Autodesk Inventor part; units mm, degrees
(part 3 of 3)
sketch "Sketch16" plane through (0, 0, 5) normal (0, 0, 1) x (1, 0, 0)
  circle A0 centre (-2.0556, -8.0514) radius 2.05 projected
  circle A1 centre (-5.9738, -25.7804) radius 2.05 projected
  circle A2 centre (11.7552, -29.6986) radius 2.05 projected
  circle A3 centre (15.6735, -11.9696) radius 2.05 projected
  circle A4 centre (-7.3556, -16.1775) radius 1.55 projected
  circle A5 centre (17.0553, -21.5725) radius 1.55 projected
  circle A6 centre (2.1523, -31.0805) radius 1.55 projected
  circle A7 centre (7.5473, -6.6695) radius 1.55 projected
  line L0 (-8.9194, -96.699) -> (-12.8137, -111.6638) projected
  arc A8 (-16.3595, -112.3464) -> (-12.8137, -111.6638) centre (-14.7493, -111.1602) ccw projected
  arc A9 (-16.3595, -112.3464) -> (-18.9305, -109.3855) centre (-36.0848, -126.8778) ccw projected
  arc A10 (-19.7333, -106.4881) -> (-18.9305, -109.3855) centre (-16.83, -107.2436) ccw projected
  line L1 (-19.7333, -106.4881) -> (-18.513, -101.7988) projected
  arc A11 (-16.9119, -99.2479) -> (-18.513, -101.7988) centre (-13.6742, -103.058) ccw projected
  arc A12 (-16.9119, -99.2479) -> (-12.3264, -94.8408) centre (-50.585, -59.6232) ccw projected
  arc A13 (-8.9194, -96.699) -> (-12.3264, -94.8408) centre (-10.8549, -96.1953) ccw projected
  arc A14 (-68.172, -108.5588) -> (-61.3963, -110.4869) centre (-50.585, -59.6232) ccw projected
  arc A15 (-60.0679, -113.4218) -> (-61.3963, -110.4869) centre (-61.8121, -112.4432) ccw projected
  arc A16 (-60.0679, -113.4218) -> (-62.0734, -117.8863) centre (-36.0848, -126.8778) ccw projected
  arc A17 (-65.5871, -118.4003) -> (-62.0734, -117.8863) centre (-63.9634, -117.2324) ccw projected
  line L2 (-65.5871, -118.4003) -> (-70.472, -111.6088) projected
  arc A18 (-68.172, -108.5588) -> (-70.472, -111.6088) centre (-68.8484, -110.441) ccw projected
  circle A19 centre (-16.1129, -136.1039) radius 2.05 projected
  circle A20 centre (-26.8587, -106.9059) radius 2.05 projected
  circle A21 centre (-56.0568, -117.6516) radius 2.05 projected
  circle A22 centre (-45.311, -146.8497) radius 2.05 projected
  circle A23 centre (-43.6086, -47.5396) radius 2.1 projected
  circle A24 centre (-50.585, -18.9546) radius 2.1 projected
  circle A25 centre (-57.5615, -47.5396) radius 2.1 projected
  circle A26 centre (-85.8051, -39.2889) radius 2.1 projected
  circle A27 centre (-64.538, -59.6232) radius 2.1 projected
  circle A28 centre (-85.8051, -79.9575) radius 2.1 projected
  circle A29 centre (-57.5615, -71.7068) radius 2.1 projected
  circle A30 centre (-50.585, -100.2918) radius 2.1 projected
  circle A31 centre (-43.6086, -71.7068) radius 2.1 projected
  circle A32 centre (-15.365, -79.9575) radius 2.1 projected
  circle A33 centre (-15.365, -39.2889) radius 2.1 projected
  circle A34 centre (-36.6321, -59.6232) radius 2.1 projected
  line L3 (-44.13, -38.9303) -> (-49.053, -44.7973) projected
  arc A35 (-52.1171, -44.7973) -> (-49.053, -44.7973) centre (-50.585, -43.5117) ccw projected
  line L4 (-52.1171, -44.7973) -> (-57.0401, -38.9303) projected
  arc A36 (-55.2842, -34.0514) -> (-57.0401, -38.9303) centre (-54.742, -37.0019) ccw projected
  arc A37 (-45.8859, -34.0514) -> (-55.2842, -34.0514) centre (-50.585, -59.6232) ccw projected
  arc A38 (-44.13, -38.9303) -> (-45.8859, -34.0514) centre (-46.4281, -37.0019) ccw projected
  line L5 (-65.2781, -43.6865) -> (-62.6586, -50.8834) projected
  arc A39 (-64.1907, -53.5371) -> (-62.6586, -50.8834) centre (-64.538, -51.5674) ccw projected
  line L6 (-64.1907, -53.5371) -> (-71.7331, -54.867) projected
  arc A40 (-75.0805, -50.9068) -> (-71.7331, -54.867) centre (-72.2541, -51.9126) ccw projected
  arc A41 (-70.3813, -42.7677) -> (-75.0805, -50.9068) centre (-50.585, -59.6232) ccw projected
  arc A42 (-65.2781, -43.6865) -> (-70.3813, -42.7677) centre (-68.0971, -44.7125) ccw projected
  line L7 (-71.7331, -64.3793) -> (-64.1907, -65.7093) projected
  arc A43 (-62.6586, -68.3629) -> (-64.1907, -65.7093) centre (-64.538, -67.6789) ccw projected
  line L8 (-62.6586, -68.3629) -> (-65.2781, -75.5599) projected
  arc A44 (-70.3813, -76.4787) -> (-65.2781, -75.5599) centre (-68.0971, -74.5338) ccw projected
  arc A45 (-75.0805, -68.3395) -> (-70.3813, -76.4787) centre (-50.585, -59.6232) ccw projected
  arc A46 (-71.7331, -64.3793) -> (-75.0805, -68.3395) centre (-72.2541, -67.3338) ccw projected
  line L9 (-57.0401, -80.316) -> (-52.1171, -74.449) projected
  arc A47 (-49.053, -74.449) -> (-52.1171, -74.449) centre (-50.585, -75.7346) ccw projected
  line L10 (-49.053, -74.449) -> (-44.13, -80.316) projected
  arc A48 (-45.8859, -85.195) -> (-44.13, -80.316) centre (-46.4281, -82.2444) ccw projected
  arc A49 (-55.2842, -85.195) -> (-45.8859, -85.195) centre (-50.585, -59.6232) ccw projected
  arc A50 (-57.0401, -80.316) -> (-55.2842, -85.195) centre (-54.742, -82.2444) ccw projected
  line L11 (-35.892, -75.5599) -> (-38.5115, -68.3629) projected
  arc A51 (-36.9794, -65.7093) -> (-38.5115, -68.3629) centre (-36.6321, -67.6789) ccw projected
  line L12 (-36.9794, -65.7093) -> (-29.437, -64.3793) projected
  arc A52 (-26.0896, -68.3395) -> (-29.437, -64.3793) centre (-28.916, -67.3338) ccw projected
  arc A53 (-30.7888, -76.4787) -> (-26.0896, -68.3395) centre (-50.585, -59.6232) ccw projected
  arc A54 (-35.892, -75.5599) -> (-30.7888, -76.4787) centre (-33.073, -74.5338) ccw projected
  line L13 (-29.437, -54.867) -> (-36.9794, -53.5371) projected
  arc A55 (-38.5115, -50.8834) -> (-36.9794, -53.5371) centre (-36.6321, -51.5674) ccw projected
  line L14 (-38.5115, -50.8834) -> (-35.892, -43.6865) projected
  arc A56 (-30.7888, -42.7677) -> (-35.892, -43.6865) centre (-33.073, -44.7125) ccw projected
  arc A57 (-26.0896, -50.9068) -> (-30.7888, -42.7677) centre (-50.585, -59.6232) ccw projected
  arc A58 (-29.437, -54.867) -> (-26.0896, -50.9068) centre (-28.916, -51.9126) ccw projected
  arc A59 (-83.4142, -91.845) -> (-62.0753, -104.165) centre (-50.585, -59.6232) ccw projected
  arc A60 (-83.0768, -85.9345) -> (-83.4142, -91.845) centre (-80.5595, -89.0431) ccw projected
  line L15 (-83.0768, -85.9345) -> (-78.075, -81.8841) projected
  arc A61 (-74.0235, -82.1373) -> (-78.075, -81.8841) centre (-76.1871, -84.2156) ccw projected
  arc A62 (-74.0235, -82.1373) -> (-58.3636, -91.1786) centre (-50.585, -59.6232) ccw projected
  arc A63 (-56.1186, -94.5607) -> (-58.3636, -91.1786) centre (-59.0817, -94.0914) ccw projected
  line L16 (-56.1186, -94.5607) -> (-57.1254, -100.9175) projected
  arc A64 (-62.0753, -104.165) -> (-57.1254, -100.9175) centre (-61.0762, -100.2918) ccw projected
  arc A65 (-39.0948, -104.165) -> (-17.7559, -91.845) centre (-50.585, -59.6232) ccw projected
  arc A66 (-44.0447, -100.9175) -> (-39.0948, -104.165) centre (-40.0939, -100.2918) ccw projected
  line L17 (-44.0447, -100.9175) -> (-45.0515, -94.5607) projected
  arc A67 (-42.8065, -91.1786) -> (-45.0515, -94.5607) centre (-42.0884, -94.0914) ccw projected
  arc A68 (-42.8065, -91.1786) -> (-27.1466, -82.1373) centre (-50.585, -59.6232) ccw projected
  arc A69 (-23.0951, -81.8841) -> (-27.1466, -82.1373) centre (-24.983, -84.2156) ccw projected
  line L18 (-23.0951, -81.8841) -> (-18.0933, -85.9345) projected
  arc A70 (-17.7559, -91.845) -> (-18.0933, -85.9345) centre (-20.6106, -89.0431) ccw projected
  arc A71 (-6.2656, -71.9432) -> (-6.2656, -47.3031) centre (-50.585, -59.6232) ccw projected
  arc A72 (-11.5529, -74.6062) -> (-6.2656, -71.9432) centre (-10.1194, -70.8719) ccw projected
  line L19 (-11.5529, -74.6062) -> (-17.5615, -72.2997) projected
  arc A73 (-19.368, -68.6644) -> (-17.5615, -72.2997) centre (-16.4864, -69.499) ccw projected
  arc A74 (-19.368, -68.6644) -> (-19.368, -50.5819) centre (-50.585, -59.6232) ccw projected
  arc A75 (-17.5615, -46.9466) -> (-19.368, -50.5819) centre (-16.4864, -49.7474) ccw projected
  line L20 (-17.5615, -46.9466) -> (-11.5529, -44.6401) projected
  arc A76 (-6.2656, -47.3031) -> (-11.5529, -44.6401) centre (-10.1194, -48.3745) ccw projected
  arc A77 (-17.7559, -27.4014) -> (-39.0948, -15.0814) centre (-50.585, -59.6232) ccw projected
  arc A78 (-18.0933, -33.3119) -> (-17.7559, -27.4014) centre (-20.6106, -30.2033) ccw projected
  line L21 (-18.0933, -33.3119) -> (-23.0951, -37.3622) projected
  arc A79 (-27.1466, -37.109) -> (-23.0951, -37.3622) centre (-24.983, -35.0308) ccw projected
  arc A80 (-27.1466, -37.109) -> (-42.8065, -28.0678) centre (-50.585, -59.6232) ccw projected
  arc A81 (-45.0515, -24.6857) -> (-42.8065, -28.0678) centre (-42.0884, -25.155) ccw projected
  line L22 (-45.0515, -24.6857) -> (-44.0447, -18.3288) projected
  arc A82 (-39.0948, -15.0814) -> (-44.0447, -18.3288) centre (-40.0939, -18.9546) ccw projected
  arc A83 (-62.0753, -15.0814) -> (-83.4142, -27.4014) centre (-50.585, -59.6232) ccw projected
  arc A84 (-57.1254, -18.3288) -> (-62.0753, -15.0814) centre (-61.0762, -18.9546) ccw projected
  line L23 (-57.1254, -18.3288) -> (-56.1186, -24.6857) projected
  arc A85 (-58.3636, -28.0678) -> (-56.1186, -24.6857) centre (-59.0817, -25.155) ccw projected
  arc A86 (-58.3636, -28.0678) -> (-74.0235, -37.109) centre (-50.585, -59.6232) ccw projected
  arc A87 (-78.075, -37.3622) -> (-74.0235, -37.109) centre (-76.1871, -35.0308) ccw projected
  line L24 (-78.075, -37.3622) -> (-83.0768, -33.3119) projected
  arc A88 (-83.4142, -27.4014) -> (-83.0768, -33.3119) centre (-80.5595, -30.2033) ccw projected
  arc A89 (-94.9045, -47.3031) -> (-94.9045, -71.9432) centre (-50.585, -59.6232) ccw projected
  arc A90 (-89.6172, -44.6401) -> (-94.9045, -47.3031) centre (-91.0507, -48.3745) ccw projected
  line L25 (-89.6172, -44.6401) -> (-83.6086, -46.9466) projected
  arc A91 (-81.8021, -50.5819) -> (-83.6086, -46.9466) centre (-84.6837, -49.7474) ccw projected
  arc A92 (-81.8021, -50.5819) -> (-81.8021, -68.6644) centre (-50.585, -59.6232) ccw projected
  arc A93 (-83.6086, -72.2997) -> (-81.8021, -68.6644) centre (-84.6837, -69.499) ccw projected
  line L26 (-83.6086, -72.2997) -> (-89.6172, -74.6062) projected
  arc A94 (-94.9045, -71.9432) -> (-89.6172, -74.6062) centre (-91.0507, -70.8719) ccw projected
  circle A95 centre (-36.0848, -126.8778) radius 16 projected
  circle A96 centre (-50.585, -59.6232) radius 8 projected
  circle A97 centre (4.8498, -18.875) radius 8 projected
  circle A98 centre (-26.0687, -154.0932) radius 1.5 projected
  circle A99 centre (-104.9663, -72.7226) radius 1.5 projected
  circle A100 centre (-102.1649, -37.0532) radius 1.5 projected
  circle A101 centre (14.3857, 5.6417) radius 1.5 projected
  circle A102 centre (13.3039, -43.7854) radius 1.5 projected
  circle A103 centre (31.1494, -18.2994) radius 1.5 projected
  circle A104 centre (-15.6668, -2.4109) radius 1.5 projected
  circle A105 centre (-91.1309, -21.0881) radius 1.5 projected
  circle A106 centre (-106.5395, -53.3794) radius 1.5 projected
  circle A107 centre (-53.3702, -150.5044) radius 1.5 projected
  circle A108 centre (-7.6073, -133.6622) radius 1.5 projected
  line L27 (-9.7265, -123.6247) -> (9.9725, -47.9268) projected
  line L28 (9.9725, -47.9268) -> (17.8509, -46.5376) projected
  line L29 (17.8509, -46.5376) -> (17.2063, -42.8816) projected
  arc A109 (17.2063, -42.8816) -> (31.6348, -22.2755) centre (4.8498, -18.875) ccw projected
  line L30 (31.6348, -22.2755) -> (35.2909, -21.6308) projected
  line L31 (35.2909, -21.6308) -> (33.9017, -13.7524) projected
  line L32 (33.9017, -13.7524) -> (27.008, -14.9679) projected
  arc A110 (27.008, -14.9679) -> (16.0998, 0.6106) centre (4.8498, -18.875) ccw projected
  line L33 (16.0998, 0.6106) -> (19.5998, 6.6727) projected
  line L34 (19.5998, 6.6727) -> (12.6716, 10.6727) projected
  line L35 (12.6716, 10.6727) -> (10.8154, 7.4577) projected
  arc A111 (10.8154, 7.4577) -> (-13.4829, 0.947) centre (4.8498, -18.875) ccw projected
  line L36 (-13.4829, 0.947) -> (-16.6979, 2.8032) projected
  line L37 (-16.6979, 2.8032) -> (-20.6979, -4.125) projected
  line L38 (-20.6979, -4.125) -> (-55.4348, -7.3477) projected
  arc A112 (-55.4348, -7.3477) -> (-76.835, -14.1568) centre (-50.585, -59.6232) ccw projected
  line L39 (-76.835, -14.1568) -> (-80.3713, -8.0318) projected
  line L40 (-80.3713, -8.0318) -> (-92.9509, -17.9357) projected
  arc A113 (-92.9509, -17.9357) -> (-96.423, -21.7867) centre (-50.585, -59.6232) ccw projected
  line L41 (-96.423, -21.7867) -> (-95.6743, -22.4047) projected
  arc A114 (-95.3624, -25.1669) -> (-95.6743, -22.4047) centre (-96.9475, -23.9472) ccw projected
  arc A115 (-95.3624, -25.1669) -> (-100.1355, -32.4754) centre (-50.585, -59.6232) ccw projected
  arc A116 (-102.79, -33.3003) -> (-100.1355, -32.4754) centre (-101.8895, -31.5145) ccw projected
  line L42 (-102.79, -33.3003) -> (-103.9829, -32.6988) projected
  arc A117 (-103.9829, -32.6988) -> (-106.5047, -38.4279) centre (-50.585, -59.6232) ccw projected
  line L43 (-106.5047, -38.4279) -> (-109.6106, -50.019) projected
  arc A118 (-109.6106, -50.019) -> (-110.2911, -56.2415) centre (-50.585, -59.6232) ccw projected
  line L44 (-110.2911, -56.2415) -> (-108.9573, -56.317) projected
  arc A119 (-107.0709, -58.3586) -> (-108.9573, -56.317) centre (-109.0704, -58.3138) ccw projected
  arc A120 (-107.0709, -58.3586) -> (-106.5915, -67.0745) centre (-50.585, -59.6232) ccw projected
  arc A121 (-108.2427, -69.3107) -> (-106.5915, -67.0745) centre (-108.5741, -67.3383) ccw projected
  line L45 (-108.2427, -69.3107) -> (-109.2001, -69.4715) projected
  arc A122 (-109.2001, -69.4715) -> (-108.1187, -74.5427) centre (-50.585, -59.6232) ccw projected
  line L46 (-108.1187, -74.5427) -> (-102.1764, -89.4094) projected
  line L47 (-102.1764, -89.4094) -> (-96.0514, -85.8732) projected
  arc A123 (-96.0514, -85.8732) -> (-93.2051, -90.2791) centre (-50.585, -59.6232) ccw projected
  line L48 (-93.2051, -90.2791) -> (-56.6733, -141.0681) projected
  arc A124 (-57.2313, -148.7428) -> (-56.6733, -141.0681) centre (-61.5442, -144.5716) ccw projected
  line L49 (-57.2313, -148.7428) -> (-59.0263, -150.5988) projected
  line L50 (-59.0263, -150.5988) -> (-54.7134, -154.77) projected
  line L51 (-54.7134, -154.77) -> (-51.8854, -154.7228) projected
  line L52 (-51.8854, -154.7228) -> (-50.3657, -153.1515) projected
  arc A125 (-48.0859, -152.7278) -> (-50.3657, -153.1515) centre (-48.9281, -154.5419) ccw projected
  arc A126 (-48.0859, -152.7278) -> (-31.6953, -155.0377) centre (-36.0848, -126.8778) ccw projected
  arc A127 (-29.5104, -156.3231) -> (-31.6953, -155.0377) centre (-31.3873, -157.0139) ccw projected
  line L53 (-29.5104, -156.3231) -> (-29.1318, -157.3516) projected
  line L54 (-29.1318, -157.3516) -> (-26.5641, -158.5378) projected
  line L55 (-26.5641, -158.5378) -> (-22.8103, -157.1563) projected
  line L56 (-22.8103, -157.1563) -> (-21.6241, -154.5886) projected
  line L57 (-21.6241, -154.5886) -> (-22.0027, -153.56) projected
  arc A128 (-21.1722, -151.1649) -> (-22.0027, -153.56) centre (-20.1257, -152.8693) ccw projected
  arc A129 (-21.1722, -151.1649) -> (-10.1895, -138.7808) centre (-36.0848, -126.8778) ccw projected
  arc A130 (-8.179, -137.6255) -> (-10.1895, -138.7808) centre (-8.3723, -139.6161) ccw projected
  line L58 (-8.179, -137.6255) -> (-6.0033, -137.8368) projected
  line L59 (-6.0033, -137.8368) -> (-3.8193, -136.0394) projected
  line L60 (-3.8193, -136.0394) -> (-3.2394, -130.0675) projected
  line L61 (-3.2394, -130.0675) -> (-5.371, -129.8605) projected
  arc A131 (-9.7265, -123.6247) -> (-5.371, -129.8605) centre (-4.8877, -124.8839) ccw projected
  circle A132 centre (4.8498, -18.875) radius 17
  circle A133 centre (-50.585, -59.6232) radius 52.5
  line L62 (-9.0369, -9.0689) -> (-30.6127, -11.0706)
  line L63 (1.764, -55.6453) -> (6.9425, -35.7457)
  point P0 (0, 0)
  point P1 (-5.9243, -32.0248)
  point P2 (-10.9161, -25.2339)
  dimension "d115" = 34
  dimension "d116" = 105
  dimension "d117" = 6
  dimension "d118" = 6
  constraints: 4 end point, 4 point on circle, 2 centre point, 2 coincident, 2 parallel
  measures "d115" diameter of A132
  measures "d116" diameter of A133
  measures "d117" distance between parallel lines of L38 L62
  measures "d118" distance between parallel lines of L27 L63
extrude "Extrusion14" cut sketch "Sketch16" against normal blind 10 contours A133 A132 L63 | A133 L62 A132
fillet "Fillet15" radius 2 6 edges at (-10.9161, -25.2339, 2.5) (-5.9243, -32.0248, 2.5) (1.764, -55.6453, 2.5) (-30.6127, -11.0706, 2.5) (-9.0369, -9.0689, 2.5) (6.9425, -35.7457, 2.5)
fillet "Fillet17" radius 2 10 edges at (-96.0514, -85.8732, 2.5) (-76.835, -14.1568, 2.5) (-20.6979, -4.125, 2.5) (-13.4829, 0.947, 2.5) (10.8154, 7.4577, 2.5) (16.0998, 0.6106, 2.5) (27.008, -14.9679, 2.5) (31.6348, -22.2755, 2.5) (17.2063, -42.8816, 2.5) (9.9725, -47.9268, 2.5)
body "Solid2"
